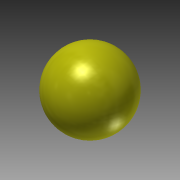
# Autodesk Inventor part: LightBulb
Saved by Autodesk Inventor 2014 SP1 (Build 180222100, 222)
## iProperties
Created: 2015-04-12
Part Number: LightBulb
Material: Rubber
Document SubType Name: Modeling
Designer: david
Density: 0.425163 g/cm^3
Appearance: Rubber - Black - Version 1.1
Mass: 57 g
Surface Area: 126.677 cm^2
Volume: 134.066 cm^3
Author: david
Autodesk Inventor part; units mm, degrees
ref_plane "YZ Plane" through (0, 0, 0) normal (1, 0, 0) x (0, 1, 0)
ref_plane "XZ Plane" through (0, 0, 0) normal (0, 1, 0) x (-1, 0, 0)
ref_plane "XY Plane" through (0, 0, 0) normal (0, 0, 1) x (1, 0, 0)
sketch "Sketch1" plane through (0, 0, 0) normal (0, 1, 0) x (-1, 0, 0)
  circle A0 centre (0, 0) radius 31.75
  line L0 (31.5833, -3.2493) -> (-31.5833, 3.2493)
  dimension "LightBulb_MinSize" = 63.5
  constraints: 2 end point, 2 point on circle, 1 centre point, 1 coincident, 1 midpoint
  measures "LightBulb_MinSize" diameter of A0
revolve "Revolution1" add sketch "Sketch1" angle 360 about axis through (-31.5833, 0, -3.2493) along (0.9947494, 0, 0.1023405) picked at (2.5389, 17.8193) contours A0 L0
body "Solid1"
